Autodesk Fusion 360 part; units mm, degrees
(part 3 of 3)
sketch "Schizzo3 (17)" plane through (0, 14, 0) normal (0, 1, 0) x (1, 0, 0) in component "12_Carter_SG90_Sinistro_removibile"
  line L0 (-69.5, -71.9) -> (-40.5, -71.9)
  line L1 (-40.5, -71.9) -> (-40.5, -93.6)
  line L2 (-40.5, -93.6) -> (-69.5, -93.6)
  line L3 (-69.5, -93.6) -> (-69.5, -71.9)
extrude "Estrusione_Parete_Anteriore_carter_Sinistro" add sketch "Schizzo3 (17)" along normal blind 2.5 bodies 25 in component "12_Carter_SG90_Sinistro_removibile"
ref_plane "Piano di lavoro4" through (0, 0, 91.1) normal (0, 0, 1) x (1, 0, 0) in component "12_Carter_SG90_Sinistro_removibile"
sketch "Schizzo4 (17)" plane through (0, 0, 91.1) normal (0, 0, 1) x (1, 0, 0) in component "12_Carter_SG90_Sinistro_removibile"
  line L0 (-69.5, -27.8) -> (-40.5, -27.8)
  line L1 (-40.5, -27.8) -> (-40.5, 16.5)
  line L2 (-40.5, 16.5) -> (-69.5, 16.5)
  line L3 (-69.5, 16.5) -> (-69.5, -27.8)
extrude "Estrusione_Tetto_carter_Sinistro" add sketch "Schizzo4 (17)" along normal blind 2.5 bodies 25 in component "12_Carter_SG90_Sinistro_removibile"
ref_plane "Piano di lavoro5" through (-69.5, 0, 0) normal (1, 0, 0) x (0, 1, 0) in component "12_Carter_SG90_Sinistro_removibile"
sketch "Schizzo5 (10)" plane through (-69.5, 0, 0) normal (1, 0, 0) x (0, 0, -1) in component "12_Carter_SG90_Sinistro_removibile"
  circle A0 centre (-81.5, -23.55) radius 1.35
extrude "Foro_M2_5_carter_Sinistro_01" cut sketch "Schizzo5 (10)" along normal blind 2.5 bodies 25 in component "12_Carter_SG90_Sinistro_removibile"
ref_plane "Piano di lavoro6" through (-69.5, 0, 0) normal (1, 0, 0) x (0, 1, 0) in component "12_Carter_SG90_Sinistro_removibile"
sketch "Schizzo6 (10)" plane through (-69.5, 0, 0) normal (1, 0, 0) x (0, 0, -1) in component "12_Carter_SG90_Sinistro_removibile"
  circle A0 centre (-81.5, 12.25) radius 1.35
extrude "Foro_M2_5_carter_Sinistro_02" cut sketch "Schizzo6 (10)" along normal blind 2.5 bodies 25 in component "12_Carter_SG90_Sinistro_removibile"
ref_plane "Piano di lavoro1" through (67, 0, 0) normal (1, 0, 0) x (0, 1, 0) in component "13_Carter_SG90_Destro_removibile"
sketch "Schizzo1 (22)" plane through (67, 0, 0) normal (1, 0, 0) x (0, 0, -1) in component "13_Carter_SG90_Destro_removibile"
  line L0 (-71.9, -27.8) -> (-93.6, -27.8)
  line L1 (-93.6, -27.8) -> (-93.6, 16.5)
  line L2 (-93.6, 16.5) -> (-71.9, 16.5)
  line L3 (-71.9, 16.5) -> (-71.9, -27.8)
extrude "Estrusione_Parete_esterna_carter_Destro" add sketch "Schizzo1 (22)" along normal blind 2.5 separate body makes body 26 in component "13_Carter_SG90_Destro_removibile"
ref_plane "Piano di lavoro2" through (0, -27.8, 0) normal (0, 1, 0) x (0, 0, 1) in component "13_Carter_SG90_Destro_removibile"
sketch "Schizzo2 (20)" plane through (0, -27.8, 0) normal (0, 1, 0) x (1, 0, 0) in component "13_Carter_SG90_Destro_removibile"
  line L0 (40.5, -71.9) -> (69.5, -71.9)
  line L1 (69.5, -71.9) -> (69.5, -93.6)
  line L2 (69.5, -93.6) -> (40.5, -93.6)
  line L3 (40.5, -93.6) -> (40.5, -71.9)
extrude "Estrusione_Parete_Posteriore_carter_Destro" add sketch "Schizzo2 (20)" along normal blind 2.5 bodies 26 in component "13_Carter_SG90_Destro_removibile"
ref_plane "Piano di lavoro3" through (0, 14, 0) normal (0, 1, 0) x (0, 0, 1) in component "13_Carter_SG90_Destro_removibile"
sketch "Schizzo3 (18)" plane through (0, 14, 0) normal (0, 1, 0) x (1, 0, 0) in component "13_Carter_SG90_Destro_removibile"
  line L0 (40.5, -71.9) -> (69.5, -71.9)
  line L1 (69.5, -71.9) -> (69.5, -93.6)
  line L2 (69.5, -93.6) -> (40.5, -93.6)
  line L3 (40.5, -93.6) -> (40.5, -71.9)
extrude "Estrusione_Parete_Anteriore_carter_Destro" add sketch "Schizzo3 (18)" along normal blind 2.5 bodies 26 in component "13_Carter_SG90_Destro_removibile"
ref_plane "Piano di lavoro4" through (0, 0, 91.1) normal (0, 0, 1) x (1, 0, 0) in component "13_Carter_SG90_Destro_removibile"
sketch "Schizzo4 (18)" plane through (0, 0, 91.1) normal (0, 0, 1) x (1, 0, 0) in component "13_Carter_SG90_Destro_removibile"
  line L0 (40.5, -27.8) -> (69.5, -27.8)
  line L1 (69.5, -27.8) -> (69.5, 16.5)
  line L2 (69.5, 16.5) -> (40.5, 16.5)
  line L3 (40.5, 16.5) -> (40.5, -27.8)
extrude "Estrusione_Tetto_carter_Destro" add sketch "Schizzo4 (18)" along normal blind 2.5 bodies 26 in component "13_Carter_SG90_Destro_removibile"
ref_plane "Piano di lavoro5" through (67, 0, 0) normal (1, 0, 0) x (0, 1, 0) in component "13_Carter_SG90_Destro_removibile"
sketch "Schizzo5 (11)" plane through (67, 0, 0) normal (1, 0, 0) x (0, 0, -1) in component "13_Carter_SG90_Destro_removibile"
  circle A0 centre (-81.5, -23.55) radius 1.35
extrude "Foro_M2_5_carter_Destro_01" cut sketch "Schizzo5 (11)" along normal blind 2.5 bodies 26 in component "13_Carter_SG90_Destro_removibile"
ref_plane "Piano di lavoro6" through (67, 0, 0) normal (1, 0, 0) x (0, 1, 0) in component "13_Carter_SG90_Destro_removibile"
sketch "Schizzo6 (11)" plane through (67, 0, 0) normal (1, 0, 0) x (0, 0, -1) in component "13_Carter_SG90_Destro_removibile"
  circle A0 centre (-81.5, 12.25) radius 1.35
extrude "Foro_M2_5_carter_Destro_02" cut sketch "Schizzo6 (11)" along normal blind 2.5 bodies 26 in component "13_Carter_SG90_Destro_removibile"
ref_plane "Piano di lavoro1" through (0, 0, 83.5) normal (0, 0, 1) x (1, 0, 0) in component "14_Guscio_mobile_cannone_removibile"
sketch "Schizzo1 (23)" plane through (0, 0, 83.5) normal (0, 0, 1) x (1, 0, 0) in component "14_Guscio_mobile_cannone_removibile"
  line L0 (-28, -13) -> (-25.5, -13)
  line L1 (-25.5, -13) -> (-25.5, 43)
  line L2 (-25.5, 43) -> (-28, 43)
  line L3 (-28, 43) -> (-28, -13)
extrude "Estrusione_Parete_mobile_Ovest" add sketch "Schizzo1 (23)" along normal blind 26 separate body makes body 27 in component "14_Guscio_mobile_cannone_removibile"
sketch "Schizzo2 (21)" plane through (0, 0, 83.5) normal (0, 0, 1) x (1, 0, 0) in component "14_Guscio_mobile_cannone_removibile"
  line L0 (-28, -13) -> (28, -13)
  line L1 (28, -13) -> (28, -10.5)
  line L2 (28, -10.5) -> (-28, -10.5)
  line L3 (-28, -10.5) -> (-28, -13)
extrude "Estrusione_Parete_mobile_Posteriore" add sketch "Schizzo2 (21)" along normal blind 26 bodies 27 in component "14_Guscio_mobile_cannone_removibile"
sketch "Schizzo3 (19)" plane through (0, 0, 83.5) normal (0, 0, 1) x (1, 0, 0) in component "14_Guscio_mobile_cannone_removibile"
  line L0 (25.5, -13) -> (28, -13)
  line L1 (28, -13) -> (28, 43)
  line L2 (28, 43) -> (25.5, 43)
  line L3 (25.5, 43) -> (25.5, -13)
extrude "Estrusione_Parete_mobile_Est" add sketch "Schizzo3 (19)" along normal blind 26 bodies 27 in component "14_Guscio_mobile_cannone_removibile"
ref_plane "Piano di lavoro2" through (0, 0, 107) normal (0, 0, 1) x (1, 0, 0) in component "14_Guscio_mobile_cannone_removibile"
sketch "Schizzo4 (19)" plane through (0, 0, 107) normal (0, 0, 1) x (1, 0, 0) in component "14_Guscio_mobile_cannone_removibile"
  line L0 (-28, -13) -> (28, -13)
  line L1 (28, -13) -> (28, 43)
  line L2 (28, 43) -> (-28, 43)
  line L3 (-28, 43) -> (-28, -13)
extrude "Estrusione_Tetto_guscio_mobile_cannone" add sketch "Schizzo4 (19)" along normal blind 2.5 bodies 27 in component "14_Guscio_mobile_cannone_removibile"
ref_plane "Piano di lavoro3" through (0, 0, 106.2) normal (0, 0, 1) x (1, 0, 0) in component "14_Guscio_mobile_cannone_removibile"
sketch "Schizzo5 (12)" plane through (0, 0, 106.2) normal (0, 0, 1) x (1, 0, 0) in component "14_Guscio_mobile_cannone_removibile"
  line L0 (-15, -13) -> (-7, -13)
  line L1 (-7, -13) -> (-7, 2)
  line L2 (-7, 2) -> (-15, 2)
  line L3 (-15, 2) -> (-15, -13)
extrude "Estrusione_Longherone_rinforzo_tasca_culatta_Ovest" add sketch "Schizzo5 (12)" along normal blind 1 bodies 27 in component "14_Guscio_mobile_cannone_removibile"
sketch "Schizzo6 (12)" plane through (0, 0, 106.2) normal (0, 0, 1) x (1, 0, 0) in component "14_Guscio_mobile_cannone_removibile"
  line L0 (7, -13) -> (15, -13)
  line L1 (15, -13) -> (15, 2)
  line L2 (15, 2) -> (7, 2)
  line L3 (7, 2) -> (7, -13)
extrude "Estrusione_Longherone_rinforzo_tasca_culatta_Est" add sketch "Schizzo6 (12)" along normal blind 1 bodies 27 in component "14_Guscio_mobile_cannone_removibile"
sketch "Schizzo7 (10)" plane through (0, 0, 106.2) normal (0, 0, 1) x (1, 0, 0) in component "14_Guscio_mobile_cannone_removibile"
  line L0 (-15, -1) -> (15, -1)
  line L1 (15, -1) -> (15, 2)
  line L2 (15, 2) -> (-15, 2)
  line L3 (-15, 2) -> (-15, -1)
extrude "Estrusione_Traversa_anteriore_rinforzo_tasca_culatta" add sketch "Schizzo7 (10)" along normal blind 1 bodies 27 in component "14_Guscio_mobile_cannone_removibile"
ref_plane "Piano di lavoro4" through (0, -13, 0) normal (0, 1, 0) x (0, 0, 1) in component "14_Guscio_mobile_cannone_removibile"
sketch "Schizzo8 (10)" plane through (0, -13, 0) normal (0, 1, 0) x (1, 0, 0) in component "14_Guscio_mobile_cannone_removibile"
  line L0 (-7, -90.5) -> (7, -90.5)
  line L1 (7, -90.5) -> (7, -109.5)
  line L2 (7, -109.5) -> (-7, -109.5)
  line L3 (-7, -109.5) -> (-7, -90.5)
extrude "Finestra_posteriore_culatta_manuale" cut sketch "Schizzo8 (10)" along normal blind 2.5 bodies 27 in component "14_Guscio_mobile_cannone_removibile"
sketch "Schizzo9 (9)" plane through (0, 0, 107) normal (0, 0, 1) x (1, 0, 0) in component "14_Guscio_mobile_cannone_removibile"
  line L0 (-7, -13) -> (7, -13)
  line L1 (7, -13) -> (7, -1)
  line L2 (7, -1) -> (-7, -1)
  line L3 (-7, -1) -> (-7, -13)
extrude "Asola_tetto_accesso_culatta_manuale" cut sketch "Schizzo9 (9)" along normal blind 2.5 bodies 27 in component "14_Guscio_mobile_cannone_removibile"
ref_plane "Piano di lavoro5" through (0, 0, 107.5) normal (0, 0, 1) x (1, 0, 0) in component "14_Guscio_mobile_cannone_removibile"
sketch "Schizzo10 (9)" plane through (0, 0, 107.5) normal (0, 0, 1) x (1, 0, 0) in component "14_Guscio_mobile_cannone_removibile"
  line L0 (-15, -13) -> (15, -13)
  line L1 (15, -13) -> (15, 2)
  line L2 (15, 2) -> (-15, 2)
  line L3 (-15, 2) -> (-15, -13)
extrude "Tasca_coperchio_culatta_a_filo" cut sketch "Schizzo10 (9)" along normal blind 2 bodies 27 in component "14_Guscio_mobile_cannone_removibile"
ref_plane "Piano di lavoro6" through (0, -6, 0) normal (0, 1, 0) x (0, 0, 1) in component "14_Guscio_mobile_cannone_removibile"
sketch "Schizzo11 (8)" plane through (0, -6, 0) normal (0, 1, 0) x (1, 0, 0) in component "14_Guscio_mobile_cannone_removibile"
  circle A0 centre (0, -96.5) radius 5.5
extrude "Estrusione_Guida_interna_culatta_manuale" add sketch "Schizzo11 (8)" along normal blind 8 separate body makes body 28 in component "14_Guscio_mobile_cannone_removibile"
ref_plane "Piano di lavoro7" through (0, -6, 0) normal (0, 1, 0) x (0, 0, 1) in component "14_Guscio_mobile_cannone_removibile"
sketch "Schizzo12 (7)" plane through (0, -6, 0) normal (0, 1, 0) x (1, 0, 0) in component "14_Guscio_mobile_cannone_removibile"
  circle A0 centre (0, -96.5) radius 4
extrude "Foro_coassiale_guida_culatta_manuale" cut sketch "Schizzo12 (7)" along normal blind 8 bodies 28 in component "14_Guscio_mobile_cannone_removibile"
ref_plane "Piano di lavoro8" through (0, 0, 100.8) normal (0, 0, 1) x (1, 0, 0) in component "14_Guscio_mobile_cannone_removibile"
sketch "Schizzo13 (7)" plane through (0, 0, 100.8) normal (0, 0, 1) x (1, 0, 0) in component "14_Guscio_mobile_cannone_removibile"
  line L0 (-2, -6) -> (2, -6)
  line L1 (2, -6) -> (2, 2)
  line L2 (2, 2) -> (-2, 2)
  line L3 (-2, 2) -> (-2, -6)
extrude "Estrusione_Nervatura_tetto_guida_culatta" add sketch "Schizzo13 (7)" along normal blind 6.4 bodies 27 28 in component "14_Guscio_mobile_cannone_removibile"
ref_plane "Piano di lavoro9" through (0, 0, 103) normal (0, 0, 1) x (1, 0, 0) in component "14_Guscio_mobile_cannone_removibile"
sketch "Schizzo14 (6)" plane through (0, 0, 103) normal (0, 0, 1) x (1, 0, 0) in component "14_Guscio_mobile_cannone_removibile"
  circle A0 centre (-10.75, -4) radius 3
extrude "Estrusione_Boss_M2_5_coperchio_culatta_01" add sketch "Schizzo14 (6)" along normal blind 4.2 bodies 27 in component "14_Guscio_mobile_cannone_removibile"
sketch "Schizzo15 (6)" plane through (0, 0, 103) normal (0, 0, 1) x (1, 0, 0) in component "14_Guscio_mobile_cannone_removibile"
  circle A0 centre (-10.75, -4) radius 1.1
extrude "Preforo_M2_5_coperchio_culatta_01" cut sketch "Schizzo15 (6)" along normal blind 4.6 bodies 27 in component "14_Guscio_mobile_cannone_removibile"
sketch "Schizzo16 (6)" plane through (0, 0, 103) normal (0, 0, 1) x (1, 0, 0) in component "14_Guscio_mobile_cannone_removibile"
  circle A0 centre (10.75, -4) radius 3
extrude "Estrusione_Boss_M2_5_coperchio_culatta_02" add sketch "Schizzo16 (6)" along normal blind 4.2 bodies 27 in component "14_Guscio_mobile_cannone_removibile"
sketch "Schizzo17 (5)" plane through (0, 0, 103) normal (0, 0, 1) x (1, 0, 0) in component "14_Guscio_mobile_cannone_removibile"
  circle A0 centre (10.75, -4) radius 1.1
extrude "Preforo_M2_5_coperchio_culatta_02" cut sketch "Schizzo17 (5)" along normal blind 4.6 bodies 27 in component "14_Guscio_mobile_cannone_removibile"
sketch "Schizzo18 (5)" plane through (0, 0, 83.5) normal (0, 0, 1) x (1, 0, 0) in component "14_Guscio_mobile_cannone_removibile"
  line L0 (-28, 40.5) -> (-5.5, 40.5)
  line L1 (-5.5, 40.5) -> (-5.5, 43)
  line L2 (-5.5, 43) -> (-28, 43)
  line L3 (-28, 43) -> (-28, 40.5)
extrude "Estrusione_Parete_mobile_Anteriore_Ovest" add sketch "Schizzo18 (5)" along normal blind 26 bodies 27 in component "14_Guscio_mobile_cannone_removibile"
sketch "Schizzo19 (4)" plane through (0, 0, 83.5) normal (0, 0, 1) x (1, 0, 0) in component "14_Guscio_mobile_cannone_removibile"
  line L0 (5.5, 40.5) -> (28, 40.5)
  line L1 (28, 40.5) -> (28, 43)
  line L2 (28, 43) -> (5.5, 43)
  line L3 (5.5, 43) -> (5.5, 40.5)
extrude "Estrusione_Parete_mobile_Anteriore_Est" add sketch "Schizzo19 (4)" along normal blind 26 bodies 27 in component "14_Guscio_mobile_cannone_removibile"
ref_plane "Piano di lavoro10" through (0, 0, 102) normal (0, 0, 1) x (1, 0, 0) in component "14_Guscio_mobile_cannone_removibile"
sketch "Schizzo20 (4)" plane through (0, 0, 102) normal (0, 0, 1) x (1, 0, 0) in component "14_Guscio_mobile_cannone_removibile"
  line L0 (-5.5, 40.5) -> (5.5, 40.5)
  line L1 (5.5, 40.5) -> (5.5, 43)
  line L2 (5.5, 43) -> (-5.5, 43)
  line L3 (-5.5, 43) -> (-5.5, 40.5)
extrude "Estrusione_Ponte_superiore_cava_U_canna" add sketch "Schizzo20 (4)" along normal blind 7.5 bodies 27 in component "14_Guscio_mobile_cannone_removibile"
ref_plane "Piano di lavoro11" through (0, -13, 0) normal (0, 1, 0) x (0, 0, 1) in component "14_Guscio_mobile_cannone_removibile"
sketch "Schizzo21 (4)" plane through (0, -13, 0) normal (0, 1, 0) x (1, 0, 0) in component "14_Guscio_mobile_cannone_removibile"
  line L0 (-3, -83.5) -> (3, -83.5)
  line L1 (3, -83.5) -> (3, -87.5)
  line L2 (3, -87.5) -> (-3, -87.5)
  line L3 (-3, -87.5) -> (-3, -83.5)
extrude "Tacca_posteriore_cavo_cannone_aperta_inferiormente" cut sketch "Schizzo21 (4)" along normal blind 2.5 bodies 27 in component "14_Guscio_mobile_cannone_removibile"
ref_plane "Piano di lavoro12" through (0, 0, 85.5) normal (0, 0, 1) x (1, 0, 0) in component "14_Guscio_mobile_cannone_removibile"
sketch "Schizzo22 (4)" plane through (0, 0, 85.5) normal (0, 0, 1) x (1, 0, 0) in component "14_Guscio_mobile_cannone_removibile"
  circle A0 centre (-20, -5) radius 5
extrude "Estrusione_Colonna_M3_guscio_mobile_01" add sketch "Schizzo22 (4)" along normal blind 21.7 bodies 27 in component "14_Guscio_mobile_cannone_removibile"
sketch "Schizzo23 (3)" plane through (0, 0, 85.5) normal (0, 0, 1) x (1, 0, 0) in component "14_Guscio_mobile_cannone_removibile"
  circle A0 centre (-20, -5) radius 1.75
extrude "Foro_M3_guscio_mobile_01" cut sketch "Schizzo23 (3)" along normal blind 24 bodies 27 in component "14_Guscio_mobile_cannone_removibile"
sketch "Schizzo24 (3)" plane through (0, 0, 85.5) normal (0, 0, 1) x (1, 0, 0) in component "14_Guscio_mobile_cannone_removibile"
  circle A0 centre (20, -5) radius 5
extrude "Estrusione_Colonna_M3_guscio_mobile_02" add sketch "Schizzo24 (3)" along normal blind 21.7 bodies 27 in component "14_Guscio_mobile_cannone_removibile"
sketch "Schizzo25 (3)" plane through (0, 0, 85.5) normal (0, 0, 1) x (1, 0, 0) in component "14_Guscio_mobile_cannone_removibile"
  circle A0 centre (20, -5) radius 1.75
extrude "Foro_M3_guscio_mobile_02" cut sketch "Schizzo25 (3)" along normal blind 24 bodies 27 in component "14_Guscio_mobile_cannone_removibile"
sketch "Schizzo26 (3)" plane through (0, 0, 85.5) normal (0, 0, 1) x (1, 0, 0) in component "14_Guscio_mobile_cannone_removibile"
  circle A0 centre (-20, 35) radius 5
extrude "Estrusione_Colonna_M3_guscio_mobile_03" add sketch "Schizzo26 (3)" along normal blind 21.7 bodies 27 in component "14_Guscio_mobile_cannone_removibile"
sketch "Schizzo27 (3)" plane through (0, 0, 85.5) normal (0, 0, 1) x (1, 0, 0) in component "14_Guscio_mobile_cannone_removibile"
  circle A0 centre (-20, 35) radius 1.75
extrude "Foro_M3_guscio_mobile_03" cut sketch "Schizzo27 (3)" along normal blind 24 bodies 27 in component "14_Guscio_mobile_cannone_removibile"
sketch "Schizzo28 (3)" plane through (0, 0, 85.5) normal (0, 0, 1) x (1, 0, 0) in component "14_Guscio_mobile_cannone_removibile"
  circle A0 centre (20, 35) radius 5
extrude "Estrusione_Colonna_M3_guscio_mobile_04" add sketch "Schizzo28 (3)" along normal blind 21.7 bodies 27 in component "14_Guscio_mobile_cannone_removibile"
sketch "Schizzo29 (3)" plane through (0, 0, 85.5) normal (0, 0, 1) x (1, 0, 0) in component "14_Guscio_mobile_cannone_removibile"
  circle A0 centre (20, 35) radius 1.75
extrude "Foro_M3_guscio_mobile_04" cut sketch "Schizzo29 (3)" along normal blind 24 bodies 27 in component "14_Guscio_mobile_cannone_removibile"
ref_plane "Piano di lavoro1" through (0, 0, 107.5) normal (0, 0, 1) x (1, 0, 0) in component "15_Coperchio_culatta_L_removibile_M2_5"
sketch "Schizzo1 (24)" plane through (0, 0, 107.5) normal (0, 0, 1) x (1, 0, 0) in component "15_Coperchio_culatta_L_removibile_M2_5"
  line L0 (-14.7, -12.7) -> (14.7, -12.7)
  line L1 (14.7, -12.7) -> (14.7, 1.7)
  line L2 (14.7, 1.7) -> (-14.7, 1.7)
  line L3 (-14.7, 1.7) -> (-14.7, -12.7)
extrude "Estrusione_Piastra_superiore_coperchio_culatta_a_filo" add sketch "Schizzo1 (24)" along normal blind 1.8 separate body makes body 29 in component "15_Coperchio_culatta_L_removibile_M2_5"
ref_plane "Piano di lavoro2" through (0, -12.7, 0) normal (0, 1, 0) x (0, 0, 1) in component "15_Coperchio_culatta_L_removibile_M2_5"
sketch "Schizzo2 (22)" plane through (0, -12.7, 0) normal (0, 1, 0) x (1, 0, 0) in component "15_Coperchio_culatta_L_removibile_M2_5"
  line L0 (-6.7, -90.8) -> (6.7, -90.8)
  line L1 (6.7, -90.8) -> (6.7, -109.2)
  line L2 (6.7, -109.2) -> (-6.7, -109.2)
  line L3 (-6.7, -109.2) -> (-6.7, -90.8)
extrude "Estrusione_Piastra_posteriore_coperchio_culatta" add sketch "Schizzo2 (22)" along normal blind 1.9 bodies 29 in component "15_Coperchio_culatta_L_removibile_M2_5"
ref_plane "Piano di lavoro3" through (0, 0, 108.1) normal (0, 0, 1) x (1, 0, 0) in component "15_Coperchio_culatta_L_removibile_M2_5"
ref_plane "Piano di lavoro4" through (0, 0, 109.3) normal (0, 0, 1) x (1, 0, 0) in component "15_Coperchio_culatta_L_removibile_M2_5"
sketch "Schizzo3 (20)" plane through (0, 0, 107.5) normal (0, 0, 1) x (1, 0, 0) in component "15_Coperchio_culatta_L_removibile_M2_5"
  circle A0 centre (-10.75, -4) radius 1.35
extrude "Foro_M2_5_coperchio_culatta_01" cut sketch "Schizzo3 (20)" along normal blind 1.8 bodies 29 in component "15_Coperchio_culatta_L_removibile_M2_5"
sketch "Schizzo4 (20)" plane through (0, 0, 108.1) normal (0, 0, 1) x (1, 0, 0) in component "15_Coperchio_culatta_L_removibile_M2_5"
  circle A0 centre (-10.75, -4) radius 1.35
sketch "Schizzo5 (13)" plane through (0, 0, 109.3) normal (0, 0, 1) x (1, 0, 0) in component "15_Coperchio_culatta_L_removibile_M2_5"
  circle A0 centre (-10.75, -4) radius 2.5
loft "Svasatura_M2_5_coperchio_culatta_01" cut profiles "Schizzo4 (20)", "Schizzo5 (13)" section 1 section 2 bodies 29 in component "15_Coperchio_culatta_L_removibile_M2_5"
sketch "Schizzo6 (13)" plane through (0, 0, 107.5) normal (0, 0, 1) x (1, 0, 0) in component "15_Coperchio_culatta_L_removibile_M2_5"
  circle A0 centre (10.75, -4) radius 1.35
extrude "Foro_M2_5_coperchio_culatta_02" cut sketch "Schizzo6 (13)" along normal blind 1.8 bodies 29 in component "15_Coperchio_culatta_L_removibile_M2_5"
sketch "Schizzo7 (11)" plane through (0, 0, 108.1) normal (0, 0, 1) x (1, 0, 0) in component "15_Coperchio_culatta_L_removibile_M2_5"
  circle A0 centre (10.75, -4) radius 1.35
sketch "Schizzo8 (11)" plane through (0, 0, 109.3) normal (0, 0, 1) x (1, 0, 0) in component "15_Coperchio_culatta_L_removibile_M2_5"
  circle A0 centre (10.75, -4) radius 2.5
loft "Svasatura_M2_5_coperchio_culatta_02" cut profiles "Schizzo7 (11)", "Schizzo8 (11)" section 1 section 2 bodies 29 in component "15_Coperchio_culatta_L_removibile_M2_5"
sketch "Schizzo1 (25)" plane through (0, 0, 0) normal (0, 1, 0) x (1, 0, 0) in component "06_Sottoassieme_coperchio_stepper_torretta"
  line L0 (0, -20) -> (0, 20)
ref_plane "Piano di lavoro1" through (0, 0, 81.5) normal (0, 0, 1) x (1, 0, 0) in component "06_Sottoassieme_coperchio_stepper_torretta"
sketch "Schizzo2 (23)" plane through (0, 0, 81.5) normal (0, 0, 1) x (1, 0, 0) in component "06_Sottoassieme_coperchio_stepper_torretta"
  line L0 (-20, 0) -> (20, 0)
component "01_Piano_inferiore_colonnine_M3_supporto_batteria_integrato" placed x (1, 0, 0) y (0, 1, 0) z (0, 0, 1) at (0, 0, 0)
component "02_Piano_superiore" placed x (1, 0, 0) y (0, 1, 0) z (0, 0, 1) at (0, 0, 0)
component "03_Guscio_laterale_continuo_carro" placed x (1, 0, 0) y (0, 1, 0) z (0, 0, 1) at (0, 0, 0)
component "05_Arduino_UNO_R4_WiFi_RIFERIMENTO_XY_quota_Z_da_definire" placed x (1, 0, 0) y (0, 1, 0) z (0, 0, 1) at (33.33, 45.71, 3)
component "06_Sottoassieme_coperchio_stepper_torretta" placed x (1, 0, 0) y (0, 1, 0) z (0, 0, 1) at (0, 0, 46)
component "01_Tetto_elettronica_removibile" placed x (1, 0, 0) y (0, 1, 0) z (0, 0, 1) at (0, 0, 0) in component "06_Sottoassieme_coperchio_stepper_torretta"
component "02A_Rondella_assiale_torretta_sostituibile" placed x (1, 0, 0) y (0, 1, 0) z (0, 0, 1) at (0, 0, 0) in component "06_Sottoassieme_coperchio_stepper_torretta"
component "02_Stepper_28BYJ48_riferimento" placed x (1, 0, 0) y (0, 1, 0) z (0, 0, 1) at (0, 0, 0) in component "06_Sottoassieme_coperchio_stepper_torretta"
component "03_Base_rotante_D100_sede_D_stepper" placed x (1, 0, 0) y (0, 1, 0) z (0, 0, 1) at (0, 0, 0) in component "06_Sottoassieme_coperchio_stepper_torretta"
component "03A_Fermaglio_anti_sollevamento_Est_M3" placed x (1, 0, 0) y (0, 1, 0) z (0, 0, 1) at (0, 0, 0) in component "06_Sottoassieme_coperchio_stepper_torretta"
component "03A_Fermaglio_anti_sollevamento_Ovest_M3" placed x (1, 0, 0) y (0, 1, 0) z (0, 0, 1) at (0, 0, 0) in component "06_Sottoassieme_coperchio_stepper_torretta"
component "03A_Fermaglio_anti_sollevamento_Nord_M3" placed x (1, 0, 0) y (0, 1, 0) z (0, 0, 1) at (0, 0, 0) in component "06_Sottoassieme_coperchio_stepper_torretta"
component "03A_Fermaglio_anti_sollevamento_Sud_M3" placed x (1, 0, 0) y (0, 1, 0) z (0, 0, 1) at (0, 0, 0) in component "06_Sottoassieme_coperchio_stepper_torretta"
component "04_Torretta_parte_fissa_azimut" placed x (1, 0, 0) y (0, 1, 0) z (0, 0, 1) at (0, 0, 0) in component "06_Sottoassieme_coperchio_stepper_torretta"
component "05_Servo_TowerPro_SG90_Sinistro_riferimento" placed x (1, 0, 0) y (0, 1, 0) z (0, 0, 1) at (0, 0, 0) in component "06_Sottoassieme_coperchio_stepper_torretta"
component "06_Servo_TowerPro_SG90_Destro_riferimento" placed x (1, 0, 0) y (0, 1, 0) z (0, 0, 1) at (0, 0, 0) in component "06_Sottoassieme_coperchio_stepper_torretta"
component "07_Barrette_removibili_M2_5_SG90_Sinistra" placed x (1, 0, 0) y (0, 1, 0) z (0, 0, 1) at (0, 0, 0) in component "06_Sottoassieme_coperchio_stepper_torretta"
component "08_Barrette_removibili_M2_5_SG90_Destra" placed x (1, 0, 0) y (0, 1, 0) z (0, 0, 1) at (0, 0, 0) in component "06_Sottoassieme_coperchio_stepper_torretta"
component "09_Torretta_parte_mobile_elevazione" placed x (1, 0, 0) y (0, 1, 0) z (0, 0, 1) at (0, 0, 0) in component "06_Sottoassieme_coperchio_stepper_torretta"
component "10_Modulo_cannone_reale_PCB_solenoide_canna" placed x (1, 0, 0) y (0, 1, 0) z (0, 0, 1) at (0, 0, 0) in component "06_Sottoassieme_coperchio_stepper_torretta"
component "11_Guscio_fisso_posteriore_torretta_removibile" placed x (1, 0, 0) y (0, 1, 0) z (0, 0, 1) at (0, 0, 0) in component "06_Sottoassieme_coperchio_stepper_torretta"
component "12_Carter_SG90_Sinistro_removibile" placed x (1, 0, 0) y (0, 1, 0) z (0, 0, 1) at (0, 0, 0) in component "06_Sottoassieme_coperchio_stepper_torretta"
component "13_Carter_SG90_Destro_removibile" placed x (1, 0, 0) y (0, 1, 0) z (0, 0, 1) at (0, 0, 0) in component "06_Sottoassieme_coperchio_stepper_torretta"
component "14_Guscio_mobile_cannone_removibile" placed x (1, 0, 0) y (0, 1, 0) z (0, 0, 1) at (0, 0, 0) in component "06_Sottoassieme_coperchio_stepper_torretta"
component "15_Coperchio_culatta_L_removibile_M2_5" placed x (1, 0, 0) y (0, 1, 0) z (0, 0, 1) at (0, 0, 0) in component "06_Sottoassieme_coperchio_stepper_torretta"
equation "piano_inf_lunghezza = 170.0 mm" comment "Piano inferiore"
equation "piano_inf_larghezza = 160.0 mm" comment "Piano inferiore"
equation "piano_inf_spessore = 3.0 mm" comment "Piano inferiore"
equation "d4 = piano_inf_spessore"
equation "distanza_piani = 40.0 mm" comment "Luce libera fra i piani"
equation "piano_sup_lunghezza = 170.0 mm" comment "Piano superiore"
equation "piano_sup_larghezza = 160.0 mm" comment "Piano superiore"
equation "piano_sup_spessore = 3.0 mm" comment "Piano superiore"
equation "colonnina_diametro = 10.0 mm" comment "Colonnine base"
equation "foro_vite_M3 = 3.2 mm" comment "Gioco vite M3"
equation "colonnina_offset_bordo = 12.0 mm" comment "Centro colonnina dal bordo"
equation "dado_M3_chiave = 5.8 mm" comment "Sede esagonale dado M3"
equation "dado_M3_profondita = 2.6 mm" comment "Profondita sede dado M3"
equation "d15 = piano_inf_spessore + distanza_piani"
equation "d17 = piano_sup_spessore"
equation "d19 = piano_inf_spessore"
equation "d21 = piano_inf_spessore + distanza_piani - dado_M3_profondita"
equation "asola_fascetta_lunghezza = 10.0 mm" comment "Asola fascetta, asse Est-Ovest"
equation "asola_fascetta_larghezza = 5.0 mm" comment "Asola fascetta, asse Sud-Nord"
equation "d25 = piano_inf_spessore"
equation "d27 = piano_inf_spessore"
equation "d29 = piano_inf_spessore"
equation "d31 = piano_inf_spessore"
equation "foro_servizio_inferiore_larghezza = 10.0 mm" comment "Foro 10x10 vicino Arduino"
equation "foro_servizio_inferiore_lunghezza = 10.0 mm" comment "Foro 10x10 vicino Arduino"
equation "foro_servizio_inferiore_centro_x = -0.5 mm" comment "Centro quasi sull'asse del carro"
equation "foro_servizio_inferiore_da_sud = 110.0 mm" comment "20 mm oltre il centro dell'ultima asola fascetta"
equation "d37 = piano_inf_spessore"
equation "d39 = piano_sup_spessore"
equation "d41 = distanza_piani"
equation "d43 = piano_inf_spessore + distanza_piani"
equation "d45 = dado_M3_profondita"
equation "d47 = piano_sup_spessore"
equation "d49 = distanza_piani"
equation "d51 = piano_inf_spessore + distanza_piani"
equation "d53 = dado_M3_profondita"
equation "d55 = piano_sup_spessore"
equation "d57 = distanza_piani"
equation "d59 = piano_inf_spessore + distanza_piani"
equation "d61 = dado_M3_profondita"
equation "d63 = piano_sup_spessore"
equation "d65 = distanza_piani"
equation "d67 = piano_inf_spessore + distanza_piani"
equation "d69 = dado_M3_profondita"
equation "apertura_arduino_larghezza = 25.0 mm" comment "Apertura superiore sopra Arduino"
equation "apertura_arduino_lunghezza = 25.0 mm" comment "Apertura superiore sopra Arduino"
equation "apertura_arduino_centro_x = 33.33 mm" comment "Centro Est-Ovest apertura Arduino"
equation "apertura_arduino_centro_y = 45.71 mm" comment "Centro Sud-Nord apertura Arduino"
equation "apertura_pacco_batteria_larghezza = 33.0 mm" comment "Apertura superiore pacco batteria PCB cannone"
equation "apertura_pacco_batteria_lunghezza = 60.0 mm" comment "Apertura superiore pacco batteria PCB cannone"
equation "apertura_pacco_batteria_centro_x = -52.5 mm" comment "Centro Est-Ovest apertura pacco batteria PCB cannone"
equation "apertura_pacco_batteria_centro_y = -15.0 mm" comment "Centro Sud-Nord apertura pacco batteria PCB cannone"
equation "d79 = piano_sup_spessore"
equation "d81 = piano_sup_spessore"
equation "foro_piano_superiore_M2_5_guscio = 2.7 mm" comment "Quattro viti M2.5x8 per trattenere il guscio inferiore"
equation "d84 = piano_sup_spessore"
equation "d86 = piano_sup_spessore"
equation "d88 = piano_sup_spessore"
equation "d90 = piano_sup_spessore"
equation "batt_vano_lunghezza = 95.0 mm" comment "Vano batteria"
equation "batt_vano_larghezza = 40.0 mm" comment "Vano batteria"
equation "batt_esterno_lunghezza = 100.0 mm" comment "Supporto batteria"
equation "batt_esterno_larghezza = 45.0 mm" comment "Supporto batteria"
equation "batt_parete_spessore = 2.5 mm" comment "Pareti laterali"
equation "batt_parete_altezza = 17.0 mm" comment "Pareti laterali"
equation "batt_apertura_cavi = 10.0 mm" comment "Passaggio cavi"
equation "d99 = piano_inf_spessore"
equation "d101 = batt_parete_altezza"
equation "d103 = batt_parete_altezza"
equation "d105 = batt_parete_altezza"
equation "d107 = batt_parete_altezza"
equation "guscio_carro_larghezza_interna = 161.0 mm" comment "Vano interno guscio carro"
equation "guscio_carro_lunghezza_interna = 171.0 mm" comment "Vano interno guscio carro"
equation "guscio_carro_larghezza_esterna = 166.0 mm" comment "Ingombro esterno guscio carro"
equation "guscio_carro_lunghezza_esterna = 176.0 mm" comment "Ingombro esterno guscio carro"
equation "guscio_carro_parete = 2.5 mm" comment "Pareti guscio removibile"
equation "guscio_carro_altezza_inferiore = 46.0 mm" comment "Da piano inferiore a sommità piano superiore"
equation "guscio_carro_gioco_lato = 0.5 mm" comment "Gioco per lato rispetto ai piani"
equation "guscio_carro_altezza_laterale_continua = 76.0 mm" comment "Parete unica senza giunzione intermedia"
equation "guscio_linguetta_M2_5_spessore = 5.0 mm" comment "Fissaggio guscio sotto il piano superiore"
equation "guscio_linguetta_M2_5_span = 14.0 mm" comment "Fissaggio guscio sotto il piano superiore"
equation "guscio_linguetta_M2_5_profondita = 13.0 mm" comment "Fissaggio guscio sotto il piano superiore"
equation "guscio_linguetta_M2_5_preforo = 2.2 mm" comment "Preforo per M2.5x8"
equation "griglia_feritoie_per_parete = 3.0 mm" comment "Numero ridotto di feritoie fronte e retro"
equation "griglia_feritoia_larghezza = 42.0 mm" comment "Ventilazione vano inferiore"
equation "griglia_feritoia_altezza = 4.0 mm" comment "Ventilazione vano inferiore"
equation "griglia_feritoia_passo_verticale = 8.0 mm" comment "Ventilazione vano inferiore"
equation "d125 = guscio_carro_altezza_laterale_continua"
equation "d127 = guscio_carro_altezza_laterale_continua"
equation "d129 = guscio_carro_altezza_laterale_continua"
equation "d131 = guscio_carro_altezza_laterale_continua"
equation "arduino_r4_lunghezza = 68.58 mm" comment "Profilo ufficiale Arduino UNO R4 WiFi"
equation "arduino_r4_larghezza = 53.34 mm" comment "Profilo ufficiale Arduino UNO R4 WiFi"
equation "arduino_r4_spessore_pcb = 1.0 mm" comment "Spessore PCB ufficiale; quota Z di montaggio non ancora definita"
equation "arduino_r4_rotazione = 90.0 deg" comment "Jack DC orientato verso Sud"
equation "arduino_r4_centro_x = 33.33 mm" comment "Posizione planimetrica Arduino"
equation "arduino_r4_centro_y = 45.71 mm" comment "Posizione planimetrica Arduino"
equation "cop_lunghezza = 176.0 mm" comment "Ingombro coperchio"
equation "cop_larghezza = 166.0 mm" comment "Ingombro coperchio"
equation "cop_parete_altezza = 30.0 mm" comment "Quota locale del tetto removibile"
equation "cop_tetto_spessore = 3.0 mm" comment "Coperchio elettronica"
equation "cop_boss_M3_diametro = 10.0 mm" comment "Accesso vite M3 dal tetto alle colonnine"
equation "cop_canale_fondo_raggio_interno = 19.0 mm" comment "Fondo liscio pista cavi tipo clock-spring"
equation "cop_canale_fondo_raggio_esterno = 40.0 mm" comment "Fondo liscio pista cavi tipo clock-spring"
equation "cop_canale_fondo_quota = 20.0 mm" comment "Quota locale fondo pista cavi"
equation "cop_canale_fondo_spessore = 3.0 mm" comment "Fondo strutturale pista cavi"
equation "cop_canale_parete_spessore = 1.5 mm" comment "Pareti lisce pista cavi"
equation "cop_canale_altezza_libera = 7.0 mm" comment "Altezza libera pista cavi"
equation "stepper_corpo_diametro = 28.0 mm" comment "Riferimento stepper"
equation "stepper_corpo_altezza = 20.0 mm" comment "Riferimento stepper"
equation "stepper_albero_diametro = 5.0 mm" comment "Riferimento stepper"
equation "stepper_albero_quota_piatto = 3.0 mm" comment "Profilo D confermato"
equation "stepper_albero_lunghezza = 9.0 mm" comment "Riferimento stepper"
equation "stepper_interasse_fori = 35.0 mm" comment "Fissaggio stepper"
equation "stepper_foro_fissaggio = 4.2 mm" comment "Fissaggio stepper"
equation "stepper_svasatura_M4_diametro = 8.4 mm" comment "Testa svasata a filo"
equation "stepper_svasatura_M4_profondita = 2.1 mm" comment "Testa svasata a filo"
equation "torre_base_diametro = 100.0 mm" comment "Adattatore rotante"
equation "torre_base_spessore = 6.0 mm" comment "Adattatore rotante"
equation "torre_sede_D_diametro = 5.4 mm" comment "Mozzo D stepper"
equation "torre_sede_D_quota_piatto = 3.2 mm" comment "Mozzo D stepper"
equation "torre_rondella_assiale_DI = 76.0 mm" comment "Appoggio assiale esterno ai cavi"
equation "torre_rondella_assiale_DE = 94.0 mm" comment "Appoggio assiale esterno ai cavi"
equation "torre_rondella_assiale_spessore = 0.8 mm" comment "Appoggio assiale esterno ai cavi"
equation "torre_rondella_sede_profondita = 0.3 mm" comment "Localizzazione rondella"
equation "torre_rondella_sede_gioco = 0.2 mm" comment "Gioco per lato sede rondella"
equation "torre_guida_fissa_RI = 34.5 mm" comment "Centraggio radiale"
equation "torre_guida_fissa_RE = 36.5 mm" comment "Centraggio radiale"
equation "torre_guida_fissa_altezza = 2.6 mm" comment "Centraggio radiale"
equation "torre_gola_gioco_radiale = 0.3 mm" comment "Gioco per lato"
equation "torre_gola_profondita = 2.5 mm" comment "Guida rotante"
equation "torre_fermaglio_gioco_verticale = 0.4 mm" comment "Anti-sollevamento"
equation "torre_fermaglio_sovrapposizione = 1.5 mm" comment "Anti-sollevamento"
equation "torre_fermaglio_foro_M3 = 3.2 mm" comment "Fermagli removibili"
equation "torre_fermaglio_spallamento_altezza = 1.5 mm" comment "Antirotazione fermagli"
equation "torre_fermaglio_spallamento_larghezza = 2.0 mm" comment "Antirotazione fermagli"
equation "torre_distanziale_telaio_altezza = 6.0 mm" comment "Evita collisione con fermagli"
equation "torre_distanziale_telaio_diametro = 10.0 mm" comment "Quattro appoggi M3"
equation "torre_fissa_larghezza = 80.0 mm" comment "Parte fissa torretta"
equation "torre_fissa_lunghezza = 70.0 mm" comment "Parte fissa torretta"
equation "torre_fissa_altezza = 50.0 mm" comment "Parte fissa torretta"
equation "torre_parete_spessore = 4.0 mm" comment "Parte fissa torretta"
equation "torre_perno_quota = 32.0 mm" comment "Asse elevazione"
equation "servo_corpo_lunghezza = 22.7 mm" comment "TowerPro SG90"
equation "servo_corpo_larghezza = 12.2 mm" comment "TowerPro SG90"
equation "servo_corpo_altezza = 27.0 mm" comment "TowerPro SG90"
equation "servo_ingombro_con_uscita = 30.3 mm" comment "TowerPro SG90"
equation "servo_alette_lunghezza_totale = 32.3 mm" comment "TowerPro SG90"
equation "servo_asse_da_estremita = 17.0 mm" comment "TowerPro SG90"
equation "servo_albero_sporgenza = 3.3 mm" comment "TowerPro SG90"
equation "servo_perno_diametro = 6.0 mm" comment "Perni servo coassiali"
equation "servo_gioco_inserimento = 0.5 mm" comment "Slitta servo"
equation "servo_supporto_parete = 2.5 mm" comment "Slitta servo"
equation "servo_supporto_ripiano = 2.5 mm" comment "Slitta servo"
equation "servo_barretta_spessore = 3.0 mm" comment "Chiusura removibile servo"
equation "servo_barretta_sovrapposizione = 3.0 mm" comment "Chiusura removibile servo"
equation "servo_foro_M2_5 = 2.7 mm" comment "Chiusura removibile servo"
equation "servo_preforo_M2_5 = 2.2 mm" comment "Slitta servo"
equation "servo_cavo_larghezza = 4.0 mm" comment "Cavo piatto SG90"
equation "servo_cavo_spessore = 1.0 mm" comment "Cavo piatto SG90"
equation "servo_uscita_cavo_larghezza = 5.0 mm" comment "Slitta SG90"
equation "servo_uscita_cavo_profondita = 2.0 mm" comment "Slitta SG90"
equation "servo_connettore_larghezza = 7.0 mm" comment "Connettore SG90"
equation "servo_connettore_spessore = 3.0 mm" comment "Connettore SG90"
equation "passaggio_comune_larghezza = 9.0 mm" comment "Passaggio connettori SG90"
equation "passaggio_comune_lunghezza = 7.0 mm" comment "Passaggio connettori SG90"
equation "passaggio_arco_raggio = 28.0 mm" comment "Guida cavi azimut"
equation "passaggio_arco_larghezza = 9.0 mm" comment "Guida cavi azimut"
equation "ansa_azimut_lunghezza_libera = 210.0 mm" comment "Fascio ordinato nel canale"
equation "asola_fascetta_cavi_lunghezza = 5.0 mm" comment "Fermacavi torretta"
equation "asola_fascetta_cavi_larghezza = 2.0 mm" comment "Fermacavi torretta"
equation "asola_fascetta_cavi_interasse = 7.0 mm" comment "Fermacavi torretta"
equation "asola_fascetta_cannone_mobile_interasse = 12.0 mm" comment "Ancoraggio ansa elevazione"
equation "fermacavo_fisso_inferiore_larghezza = 18.0 mm" comment "Scarico trazione sotto uscita"
equation "fermacavo_fisso_inferiore_lunghezza = 12.0 mm" comment "Scarico trazione sotto uscita"
equation "fermacavo_fisso_inferiore_spessore = 2.0 mm" comment "Scarico trazione sotto uscita"
equation "fermacavo_fisso_asole_offset_x = 1.5 mm" comment "Sposta le asole fuori dal bordo anulare"
equation "fermacavo_fisso_ponte_larghezza = 20.0 mm" comment "Ponte strutturale verso il fondo anulare"
equation "fermacavo_fisso_ponte_lunghezza = 4.0 mm" comment "Ponte strutturale verso il fondo anulare"
equation "cannone_connettore_larghezza = 5.0 mm" comment "Connettore cannone"
equation "cannone_connettore_spessore = 3.0 mm" comment "Connettore cannone"
equation "cannone_passaggio_mobile_larghezza = 6.0 mm" comment "Passaggio sotto culla"
equation "cannone_passaggio_mobile_lunghezza = 4.0 mm" comment "Passaggio sotto culla"
equation "pcb_cannone_lunghezza = 50.0 mm" comment "PCB mobile cannone"
equation "pcb_cannone_larghezza = 50.0 mm" comment "PCB mobile cannone"
equation "pcb_cannone_spessore = 2.0 mm" comment "PCB mobile cannone"
equation "pcb_cannone_foro = 3.5 mm" comment "Fori PCB cannone"
equation "pcb_cannone_foro_bordo_x = 5.0 mm" comment "Fori PCB cannone"
equation "pcb_cannone_foro_bordo_y = 5.0 mm" comment "Fori PCB cannone"
equation "solenoide_diametro = 20.0 mm" comment "Zona solenoide"
equation "solenoide_lunghezza = 25.0 mm" comment "Zona solenoide"
equation "canna_diametro_esterno = 10.0 mm" comment "Canna tubolare"
equation "canna_diametro_interno = 8.0 mm" comment "Canna tubolare"
equation "canna_parete = 1.0 mm" comment "Canna tubolare"
equation "canna_sporgenza = 46.0 mm" comment "Canna tubolare"
equation "modulo_cannone_altezza = 23.0 mm" comment "Modulo mobile"
equation "culatta_proiettile_diametro_max_provvisorio = 7.0 mm" comment "Solo proiettile morbido e inerte"
equation "culatta_proiettile_lunghezza_max_provvisoria = 10.0 mm" comment "Ingombro di caricamento da verificare"
equation "culatta_guida_diametro_esterno = 11.0 mm" comment "Invito interno coassiale"
equation "culatta_guida_diametro_interno = 8.0 mm" comment "Invito interno coassiale"
equation "culatta_guida_lunghezza = 8.0 mm" comment "Invito interno coassiale"
equation "culatta_finestra_posteriore_larghezza = 14.0 mm" comment "Apertura a L removibile"
equation "culatta_asola_tetto_lunghezza = 12.0 mm" comment "Apertura a L removibile"
equation "culatta_coperchio_larghezza = 30.0 mm" comment "Coperchio a filo removibile"
equation "culatta_coperchio_lunghezza = 15.0 mm" comment "Coperchio a filo removibile"
equation "culatta_tasca_profondita = 2.0 mm" comment "Alloggiamento coperchio removibile"
equation "culatta_coperchio_spessore = 1.8 mm" comment "Coperchio a filo removibile"
equation "culatta_coperchio_gioco_verticale = 0.2 mm" comment "Coperchio leggermente ribassato"
equation "culatta_rinforzo_locale_spessore = 0.8 mm" comment "Rinforzo a U sotto la tasca"
equation "culatta_interasse_M2_5 = 21.5 mm" comment "Due viti accessibili dall'alto"
equation "culatta_foro_M2_5 = 2.7 mm" comment "Coperchio removibile"
equation "culatta_preforo_M2_5 = 2.2 mm" comment "Boss sotto il tetto"
equation "cannone_elevazione_min = -10.0 deg" comment "Limite proposto asse elevazione"
equation "cannone_elevazione_max = 35.0 deg" comment "Limite proposto asse elevazione"
equation "passaggio_arco_angolo_iniziale = 0.0 deg" comment "Inizio guida cavi di azimut"
equation "passaggio_arco_corsa = 360.0 deg" comment "Corsa totale guida cavi di azimut"
equation "torretta_azimut_min = -180.0 deg" comment "Limite software e giunto Fusion"
equation "torretta_azimut_max = 180.0 deg" comment "Limite software e giunto Fusion"
equation "d302 = cop_parete_altezza"
equation "d304 = cop_tetto_spessore"
equation "d322 = cop_parete_altezza"
equation "d328 = cop_tetto_spessore"
equation "d330 = cop_tetto_spessore"
equation "d332 = cop_tetto_spessore"
equation "d334 = cop_tetto_spessore"
equation "d338 = cop_tetto_spessore"
equation "d342 = cop_tetto_spessore"
equation "d346 = cop_tetto_spessore"
equation "d358 = cop_canale_fondo_spessore"
equation "d360 = cop_canale_fondo_spessore"
equation "d372 = cop_tetto_spessore"
equation "d406 = stepper_corpo_altezza"
equation "d414 = stepper_albero_lunghezza"
equation "d416 = stepper_albero_lunghezza"
equation "d420 = torre_base_spessore"
equation "d422 = torre_base_spessore"
equation "d424 = torre_base_spessore"
equation "d426 = torre_base_spessore"
equation "d434 = torre_base_spessore"
equation "d438 = torre_base_spessore"
equation "d442 = torre_base_spessore"
equation "d446 = torre_base_spessore"
equation "d450 = torre_base_spessore"
equation "d626 = servo_corpo_altezza"
equation "d630 = servo_albero_sporgenza"
equation "d634 = servo_corpo_altezza"
equation "d638 = servo_albero_sporgenza"
equation "d642 = servo_barretta_spessore"
equation "d646 = servo_barretta_spessore"
equation "d650 = servo_barretta_spessore"
equation "d654 = servo_barretta_spessore"
equation "d658 = servo_barretta_spessore"
equation "d662 = servo_barretta_spessore"
equation "d666 = servo_barretta_spessore"
equation "d670 = servo_barretta_spessore"
equation "d716 = pcb_cannone_spessore"
equation "d718 = pcb_cannone_spessore"
equation "d720 = pcb_cannone_spessore"
equation "d722 = pcb_cannone_spessore"
equation "d724 = pcb_cannone_spessore"
equation "d732 = solenoide_lunghezza"
equation "d736 = solenoide_lunghezza"
equation "d740 = canna_sporgenza"
equation "d744 = canna_sporgenza"
equation "guscio_torretta_parete = 2.5 mm" comment "Gusci removibili torretta"
equation "guscio_torretta_gioco = 0.5 mm" comment "Gioco attorno a telaio, servo e modulo mobile"
equation "guscio_cannone_foro_canna = 11.0 mm" comment "Passaggio canna nel guscio mobile"
named bodies: "Piano_inferiore_colonnine_M3_supporto_batteria_integrato", "Piano_superiore", "Guscio_laterale_continuo_166x176_Z0_Z76_griglie_fronte_retro", "Tetto_fisso_canale_cavi_guida_radiale_supporto_stepper_boss_M3", "Rondella_assiale_DI76_DE94_spessore_0_8", "Corpo_stepper", "Base_rotante_D100_sede_D_gola_guida_passaggio_cavi", "Piede_fermaglio_Est", "Piede_fermaglio_Ovest", "Piede_fermaglio_Nord", "Piede_fermaglio_Sud", "Base_parte_fissa", "Corpo_SG90_Sinistro", "Corpo_SG90_Destro", "Barretta_Sinistra_01", "Barretta_Sinistra_02", "Barretta_Destra_01", "Barretta_Destra_02", "Piastra_culla_mobile", "PCB_modulo_cannone_50x50", "Appoggio_solenoide_su_PCB", "Corpo_solenoide_riferimento", "Canna_tubolare_esterna", "Parete_posteriore_guscio_torretta", "Parete_esterna_carter_Sinistro", "Parete_esterna_carter_Destro", "Parete_mobile_Ovest", "Guida_interna_culatta_manuale", "Piastra_superiore_coperchio_culatta_a_filo"
